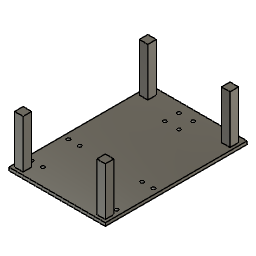
Partie_basse_imprimable.f3d v1 (Autodesk Fusion 360 design; units mm, degrees)
Autodesk Fusion 360 part; units mm, degrees
sketch "Esquisse1" plane through (0, 0, 0) normal (0, 0, 1) x (1, 0, 0)
  line L0 (-80, 100) -> (90, 100)
  line L1 (90, 100) -> (90, -150)
  line L2 (90, -150) -> (-80, -150)
  line L3 (-80, -150) -> (-80, 100)
  constraint horizontal L0
  constraint vertical L1
  constraint horizontal L2
  constraint vertical L3
extrude "Extrusion1" add sketch "Esquisse1" along normal blind 3.5
form "Forme1" [no effect]
sketch "sketch 467" plane through (0, 0, 3.5) normal (0, 0, 1) x (-1, 0, 0)
  line L0 (80, 150) -> (-90, 150)
  line L1 (-90, 150) -> (-90, -100)
  line L2 (-90, -100) -> (80, -100)
  line L3 (80, -100) -> (80, 150)
  line L4 (-70, 125) -> (-85, 125)
  line L5 (-85, 125) -> (-85, 140)
  line L6 (-85, 140) -> (-70, 140)
  line L7 (-70, 140) -> (-70, 125)
  line L8 (75, 125) -> (60, 125)
  line L9 (60, 125) -> (60, 140)
  line L10 (60, 140) -> (75, 140)
  line L11 (75, 140) -> (75, 125)
  line L12 (75, -90) -> (60, -90)
  line L13 (60, -90) -> (60, -75)
  line L14 (60, -75) -> (75, -75)
  line L15 (75, -75) -> (75, -90)
  line L16 (-85, -90) -> (-70, -90)
  line L17 (-70, -90) -> (-70, -75)
  line L18 (-70, -75) -> (-85, -75)
  line L19 (-85, -75) -> (-85, -90)
  constraint horizontal L4
  constraint vertical L5
  constraint horizontal L6
  constraint vertical L7
  constraint horizontal L8
  constraint vertical L9
  constraint horizontal L10
  constraint vertical L11
  constraint horizontal L12
  constraint vertical L13
  constraint horizontal L14
  constraint vertical L15
  constraint horizontal L16
  constraint vertical L17
  constraint horizontal L18
  constraint vertical L19
extrude "Extrusion2" add sketch "sketch 467" along normal blind 85 contours L12 L13 L14 L15 | L16 L17 L18 L19
sketch "Esquisse2" plane through (0, 0, 3.5) normal (0, 0, 1) x (-1, 0, 0)
  line L0 (-85, -75) -> (-70, -75)
  line L1 (-70, -75) -> (-70, -90)
  line L2 (-70, -90) -> (-85, -90)
  line L3 (-85, -90) -> (-85, -75)
  line L4 (75, -75) -> (75, -90)
  line L5 (75, -90) -> (60, -90)
  line L6 (60, -90) -> (60, -75)
  line L7 (60, -75) -> (75, -75)
  line L8 (80, 150) -> (-90, 150)
  line L9 (-90, 150) -> (-90, -100)
  line L10 (-90, -100) -> (80, -100)
  line L11 (80, -100) -> (80, 150)
  line L12 (75, 130) -> (60, 130)
  line L13 (60, 130) -> (60, 145)
  line L14 (60, 145) -> (75, 145)
  line L15 (75, 145) -> (75, 130)
  line L16 (-85, 130) -> (-70, 130)
  line L17 (-70, 130) -> (-70, 145)
  line L18 (-70, 145) -> (-85, 145)
  line L19 (-85, 145) -> (-85, 130)
  constraint horizontal L12
  constraint vertical L13
  constraint horizontal L14
  constraint vertical L15
  constraint horizontal L16
  constraint vertical L17
  constraint horizontal L18
  constraint vertical L19
extrude "Extrusion3" add sketch "Esquisse2" along normal blind 85 contours L12 L13 L14 L15 | L16 L17 L18 L19
sketch "Esquisse5" plane through (-60, 0, 0) normal (1, 0, 0) x (0, 1, 0)
  line L0 (-145, 3.5) -> (-130, 3.5)
  line L1 (-130, 3.5) -> (-130, 88.5)
  line L2 (-130, 88.5) -> (-145, 88.5)
  line L3 (-145, 88.5) -> (-145, 3.5)
  line L4 (-145, 88.5) -> (-130, 88.5)
  line L5 (-130, 88.5) -> (-130, 85)
  line L6 (-130, 85) -> (-145, 85)
  line L7 (-145, 85) -> (-145, 88.5)
  constraint horizontal L4
  constraint vertical L5
  constraint horizontal L6
  constraint vertical L7
  constraint coincident L2.end L3.start
move_face "DécalerLesFaces1" offset 2 1 faces at (-23.3333, -66.6667, 0)
move_body "Move1" bodies 1 to x (1, 0, 0) y (0, 1, 0) z (0, 0, 1) at (0, 0, 40)
sketch "Esquisse51" plane through (0, 0, 38) normal (0, 0, -1) x (1, 0, 0)
  line L0 (-80, 150) -> (-80, -100)
  line L1 (-80, -100) -> (90, -100)
  line L2 (90, -100) -> (90, 150)
  circle A0 centre (-12.5, -57.5) radius 3
  circle A1 centre (12.5, -57.5) radius 3
  circle A2 centre (12.5, -82.5) radius 3
  circle A3 centre (-12.5, -82.5) radius 3
  line L3 (90, 150) -> (-80, 150)
  dimension "d131" = 6
  dimension "d132" = 6
  dimension "d133" = 6
  dimension "d134" = 6
  measures "d131" diameter of A0
  measures "d132" diameter of A1
  measures "d133" diameter of A2
  measures "d134" diameter of A3
extrude "Extrusion50" cut sketch "Esquisse51" against normal blind 6 contours A0 | A1 | A2 | A3
sketch "Esquisse52" plane through (0, 0, 38) normal (0, 0, -1) x (1, 0, 0)
  circle A0 centre (-12.5, -82.5) radius 3
  circle A1 centre (-12.5, -57.5) radius 3
  circle A2 centre (12.5, -82.5) radius 3
  circle A3 centre (12.5, -57.5) radius 3
  line L0 (-80, 150) -> (-80, -100)
  line L1 (-80, -100) -> (90, -100)
  line L2 (90, -100) -> (90, 150)
  circle A4 centre (-70, 120) radius 3
  circle A5 centre (-50, 120) radius 3
  circle A6 centre (60, 120) radius 3
  circle A7 centre (80, 120) radius 3
  circle A8 centre (-50, 55) radius 3
  circle A9 centre (-70, 55) radius 3
  circle A10 centre (60, 55) radius 3
  circle A11 centre (80, 55) radius 3
  line L3 (90, 150) -> (-80, 150)
  dimension "d137" = 6
  dimension "d138" = 6
  dimension "d139" = 6
  dimension "d140" = 6
  dimension "d141" = 6
  dimension "d142" = 6
  dimension "d143" = 6
  dimension "d144" = 6
  measures "d137" diameter of A4
  measures "d138" diameter of A5
  measures "d139" diameter of A6
  measures "d140" diameter of A7
  measures "d141" diameter of A8
  measures "d142" diameter of A9
  measures "d143" diameter of A10
  measures "d144" diameter of A11
extrude "Extrusion51" cut sketch "Esquisse52" against normal blind 6 contours A4 | A5 | A6 | A7 | A8 | A9 | A10 | A11
